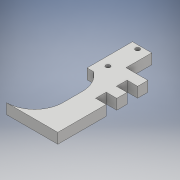
# Autodesk Inventor part: CenterFinger
Saved by Autodesk Inventor 2017 (Build 210142000, 142)
## iProperties
Created: 2017-05-09
Part Number: CenterFinger
Material: Generic
Document SubType Name: Modeling
Designer: s4461999
Density: 1 g/cm^3
Appearance: Default
Author: s4461999
Autodesk Inventor part; units mm, degrees
ref_plane "YZ Plane" through (0, 0, 0) normal (1, 0, 0) x (0, 1, 0)
ref_plane "XZ Plane" through (0, 0, 0) normal (0, 1, 0) x (-1, 0, 0)
ref_plane "XY Plane" through (0, 0, 0) normal (0, 0, 1) x (1, 0, 0)
sketch "Sketch1" plane through (0, 0, 0) normal (0, 0, 1) x (1, 0, 0)
  arc A0 (0, 0) -> (22, 22) centre (0, 22) ccw
  line L0 (22, 22) -> (22, 37)
  arc A1 (22, 37) -> (13, 54.7482) centre (0, 37) ccw
  line L1 (13, 54.7482) -> (13, 54.7482)
  line L2 (8, 90) -> (23, 90)
  line L3 (40, 62) -> (31.8, 62)
  line L4 (31.8, 62) -> (31.8, 53.8)
  line L5 (31.8, 53.8) -> (40, 53.8)
  line L6 (40, 45.8) -> (31.8, 45.8)
  line L7 (31.8, 45.8) -> (31.8, 37.6)
  line L8 (31.8, 37.6) -> (40, 37.6)
  line L9 (40, 53.8) -> (40, 45.8)
  line L10 (40, 37.6) -> (40, 0)
  line L11 (40, 62) -> (40, 70)
  line L12 (40, 70) -> (23, 70)
  line L13 (23, 70) -> (23, 90)
  line L14 (8, 90) -> (8, 54.7482)
  line L15 (8, 54.7482) -> (13, 54.7482)
  line L16 (0, 0) -> (40, 0)
  point P0 (40, 66)
  dimension "d0" = 22
  dimension "d1" = 90
  dimension "d2" = 0
  dimension "d3" = 15
  dimension "d4" = 0
  dimension "d5" = 13
  dimension "d6" = 22
  dimension "d7" = 0
  dimension "d14" = 8.2
  dimension "d15" = 8.2
  dimension "d32" = 8
  dimension "d34" = 8
  dimension "d35" = 8
  dimension "d37" = 15
  dimension "d39" = 40
  dimension "d40" = 0
  dimension "d41" = 0
  dimension "d42" = 20
  dimension "d43" = 8.2
  dimension "d44" = 90
  constraints: 34 end point, 6 perpendicular, 6 vertical, 4 point on circle, 3 horizontal, 3 parallel, 2 centre point, 2 point on line, 1 coincident, 1 midpoint
  measures "d0" radius of A0
  measures "d2" horizontal distance of point (0, 0) A0.centre
  measures "d3" distance of L0.start L0.end
  measures "d4" horizontal distance of point (0, 0) A1.centre
  measures "d5" horizontal distance of A1.centre L1.start
  measures "d6" radius of A1
  measures "d7" distance of L1.start L1.end
  measures "d14" distance between parallel lines of L5 L3
  measures "d15" distance between parallel lines of L8 L6
  measures "d32" distance of L5.end L6.start
  measures "d34" distance from line of L14 point (0, 0)
  measures "d35" distance between parallel lines of L12 L3
  measures "d37" distance between parallel lines of L13 L14
  measures "d39" distance from line of point (0, 0) L11
  measures "d40" distance between parallel lines of L9 L10
  measures "d41" distance between parallel lines of L11 L10
  measures "d42" distance between parallel lines of L12 L2
  measures "d43" distance between parallel lines of L9 L4
  measures "d44" distance between parallel lines of L16 L2
extrude "Extrusion2" add sketch "Sketch1" along normal blind 8
sketch "Sketch5" plane through (0, 0, 8) normal (0, 0, 1) x (1, 0, 0)
  line L0 (23, 90) -> (8, 90) projected
  line L1 (23, 70) -> (23, 90) projected
  point P0 (0, 0)
  point P1 (15, 87)
  point P2 (15, 64)
  dimension "d47" = 23
  dimension "d48" = 3
  dimension "d49" = 0
  dimension "d58" = 15
  measures "d47" distance of point (15, 64) point (15, 87)
  measures "d48" distance from line of L0 point (15, 87)
  measures "d49" horizontal distance of point (15, 87) point (15, 64)
  measures "d58" horizontal distance of point (0, 0) point (15, 64)
hole "Hole2" at (15, 87, 8) at (15, 64, 8) direction (0, 0, -1) diameter 3.4 end through all
body "Solid2"
